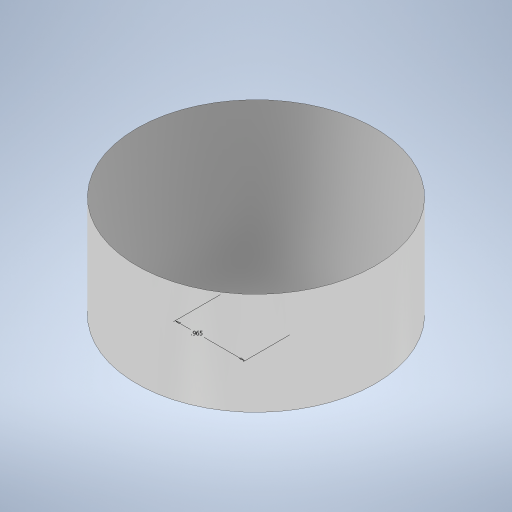
# Autodesk Inventor part: UpstreamVolume
Saved by Autodesk Inventor 2023 (Build 270158000, 158)
## iProperties
Created: 2023-01-27
Part Number: UpstreamVolume
Material: Nickel-Copper Alloy 400
Document SubType Name: Modeling
Designer: remidm
Density: 8.83 g/cm^3
Appearance: Chrome - Polished
Mass: 310.638 g
Surface Area: 352.997 cm^2
Volume: 35.1799 cm^3
DistanceBetweenHolesSweep: 0.965 in
SampleVolumeInnerHeight: 1.260 in
Author: remidm
Autodesk Inventor part; units mm, degrees
ref_plane "YZ Plane" through (0, 0, 0) normal (1, 0, 0) x (0, 1, 0)
ref_plane "XZ Plane" through (0, 0, 0) normal (0, 1, 0) x (-1, 0, 0)
ref_plane "XY Plane" through (0, 0, 0) normal (0, 0, 1) x (1, 0, 0)
sketch "Sketch1" plane through (0, 0, 0) normal (0, 0, 1) x (1, 0, 0)
  line L0 (-40, 0) -> (-40, 32)
  line L1 (-42, 34) -> (-42, -2)
  line L2 (-40, 0) -> (0, 0)
  line L3 (0, 0) -> (0, -2)
  line L4 (0, -2) -> (-42, -2)
  line L5 (0, -10.8) -> (0, 50.8) projected
  line L6 (-42, 34) -> (0, 34)
  line L7 (-40, 32) -> (0, 32)
  line L8 (0, 32) -> (0, 34)
  dimension "d5" = 2
  dimension "radius" = 40
  dimension "d7" = 2
  dimension "d37" = 2
  dimension "SampleVolumeInnerHeight" = 32
  constraints: 16 end point, 4 perpendicular, 2 point on line, 1 collinear, 1 horizontal, 1 vertical
  measures "d5" distance between parallel lines of L4 L2
  measures "radius" distance from line of L2.end L0
  measures "d7" distance between parallel lines of L0 L1
  measures "d37" distance between parallel lines of L6 L7
  measures "SampleVolumeInnerHeight" distance between parallel lines of L7 L2
revolve "Revolution1" add sketch "Sketch1" angle 360 about axis through (0, -10, 0) along (0, 1, 0) contours L2 L3 L4 L1 L6 L5 L7 L0
sketch "Sketch3" plane through (0, -2, 0) normal (0, -1, 0) x (1, 0, 0)
  line L0 (-12.4915, 0) -> (12.0084, 0)
  point P0 (0, 0)
  dimension "DistanceBetweenHolesSweep" = 24.5
  constraints: 2 end point, 1 horizontal
  measures "DistanceBetweenHolesSweep" distance of L0.end L0.start
hole "Hole2" at (0, -2, 0) direction (0, 1, 0) diameter 5.08 depth 2
hole "Hole3" at (-12.4915, -2, 0) at (12.0084, -2, 0) direction (0, 1, 0) diameter 5 depth 2
equation "\"d5\" = thickness"
equation "\"radius\" = 0.5 * SaltDiameter"
equation "\"d7\" = thickness"
equation "\"d37\" = crucible_thickness"
equation "\"SampleVolumeInnerHeight\" = 4 * SaltThickness"
equation "\"d22\" = fixation_holes_diameter"
equation "\"d30\" = PenetrationOuterDiameter"
equation "\"thickness\" = crucible_thickness"
equation "\"SaltDiameter\" = 80"
equation "\"crucible_thickness\" = 2"
equation "\"SaltThickness\" = 8"
equation "\"fixation_holes_diameter\" = 5.08"
equation "\"PenetrationOuterDiameter\" = 5"
body "Solid1"
